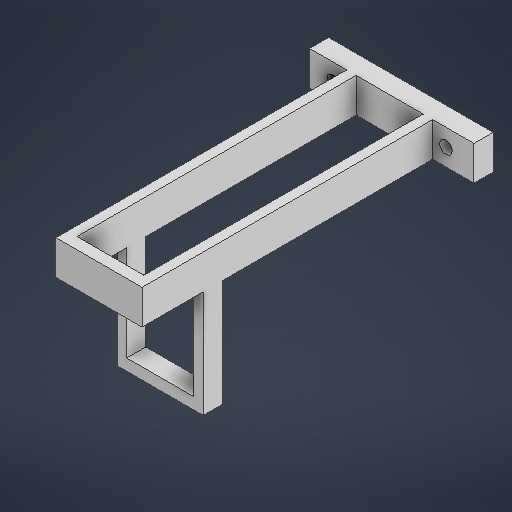
# Autodesk Inventor part: Batteryholder1
Saved by Autodesk Inventor 2026.1 (Build 301233020, 233B)
## iProperties
Created: 2025-12-01
Part Number: Batteryholder1
Material: Generic
Document SubType Name: Modeling
Designer: osama
Density: 1 g/cm^3
Appearance: Default
Author: osama
Autodesk Inventor part; units mm, degrees
ref_plane "YZ Plane" through (0, 0, 0) normal (1, 0, 0) x (0, 1, 0)
ref_plane "XZ Plane" through (0, 0, 0) normal (0, 1, 0) x (-1, 0, 0)
ref_plane "XY Plane" through (0, 0, 0) normal (0, 0, 1) x (1, 0, 0)
sketch "Sketch1" plane through (0, 0, 0) normal (0, 0, 1) x (1, 0, 0)
  line L0 (0, 0) -> (43, 0)
  line L1 (43, 0) -> (43, 9)
  line L2 (43, 9) -> (0, 9)
  line L3 (0, 9) -> (0, 0)
  dimension "d0" = 43
  dimension "d1" = 9
  constraints: 8 end point, 2 parallel, 1 horizontal, 1 perpendicular
  measures "d0" distance of L2.end L1.end
  measures "d1" distance of L1.end L0.end
extrude "Extrusion1" add sketch "Sketch1" along normal blind 5
sketch "Sketch2" plane through (0, 0, 5) normal (0, 0, 1) x (1, 0, 0)
  line L0 (43, 0) -> (43, 9) projected
  line L1 (43, 9) -> (0, 9) projected
  point P0 (0, 0)
  point P1 (35.7, 4.5)
  point P2 (6.2, 4.5)
  dimension "d11" = 7.3
  dimension "d12" = 29.5
  dimension "d13" = 4.5
  dimension "d14" = 4.5
  measures "d11" distance from line of point (35.7, 4.5) L0
  measures "d12" distance of point (35.7, 4.5) point (6.2, 4.5)
  measures "d13" distance from line of L1 point (6.2, 4.5)
  measures "d14" distance from line of L1 point (35.7, 4.5)
hole "Hole1" at (35.7, 4.5, 5) at (6.2, 4.5, 5) direction (0, 0, -1) diameter 3.3 end through all
sketch "Sketch3" plane through (0, 0, 5) normal (0, 0, 1) x (1, 0, 0)
  line L0 (0, 0) -> (43, 0) projected
  line L1 (43, 9) -> (0, 9) projected
  line L2 (9.7, 0) -> (12.2, 0)
  line L3 (12.2, 0) -> (12.2, 9)
  line L4 (12.2, 9) -> (9.7, 9)
  line L5 (9.7, 9) -> (9.7, 0)
  line L6 (29.7, 9) -> (32.2, 9)
  line L7 (32.2, 9) -> (32.2, 0)
  line L8 (32.2, 0) -> (29.7, 0)
  line L9 (29.7, 0) -> (29.7, 9)
  circle A0 centre (35.7, 4.5) radius 1.65 projected
  point P0 (29.7, 4.5)
  point P1 (12.2, 4.5)
  point P2 (32.2, 4.5)
  point P3 (29.7, 9)
  point P4 (29.7, 0)
  point P5 (32.2, 0)
  point P6 (32.2, 9)
  point P7 (12.2, 0)
  dimension "d15" = 2.5
  dimension "d16" = 2.5
  dimension "d17" = 17.5
  dimension "d18" = 3.5
  constraints: 16 end point, 4 parallel, 4 point on line, 3 midpoint, 2 horizontal, 2 perpendicular
  measures "d15" distance of L4.end L3.end
  measures "d16" distance of L7.end L8.end
  measures "d17" distance of point (29.7, 4.5) point (12.2, 4.5)
  measures "d18" distance of A0.centre point (32.2, 4.5)
extrude "Extrusion2" add sketch "Sketch3" along normal blind 76 contours L5 L1 L3 L0 | L9 L1 L7 L0
sketch "Sketch4" plane through (0, 0, 81) normal (0, 0, 1) x (1, 0, 0)
  line L0 (12.2, 9) -> (9.7, 9) projected
  line L1 (32.2, 0) -> (9.7, 0)
  line L2 (9.7, 0) -> (9.7, 9)
  line L3 (9.7, 9) -> (32.2, 9)
  line L4 (32.2, 9) -> (32.2, 0)
  point P0 (0, 0)
  constraints: 8 end point, 2 parallel, 1 horizontal, 1 perpendicular
extrude "Extrusion3" add sketch "Sketch4" against normal blind 3
sketch "Sketch7" plane through (0, 0, 0) normal (0, -1, 0) x (1, 0, 0)
  line L0 (9.7, 60) -> (9.7, 65) projected
  line L1 (9.7, 65) -> (12.2, 65)
  line L2 (12.2, 65) -> (12.2, 60)
  line L3 (12.2, 60) -> (9.7, 60)
  line L4 (9.7, 60) -> (9.7, 65)
  line L5 (32.2, 65) -> (29.7, 65) projected
  line L6 (29.7, 65) -> (32.2, 65)
  line L7 (32.2, 65) -> (32.2, 60)
  line L8 (32.2, 60) -> (29.7, 60)
  line L9 (29.7, 60) -> (29.7, 65)
  point P0 (0, 0)
  dimension "d31" = 2.5
  dimension "d32" = 5
  constraints: 16 end point, 4 parallel, 2 horizontal, 2 perpendicular, 1 point on line
  measures "d31" distance of L2.end L3.end
  measures "d32" distance of L1.end L2.end
extrude "Extrusion6" add sketch "Sketch7" along normal blind 28
sketch "Sketch8" plane through (29.7, 0, 5) normal (-1, 0, 0) x (0, 0, 1)
  line L0 (60, 0) -> (60, -28) projected
  line L1 (60, -28) -> (55, -28)
  line L2 (55, -28) -> (55, -25)
  line L3 (55, -25) -> (60, -25)
  line L4 (60, -25) -> (60, -28)
  point P0 (-5, 0)
  dimension "d35" = 5
  dimension "d36" = 3
  constraints: 8 end point, 2 parallel, 1 horizontal, 1 perpendicular
  measures "d35" distance of L2.end L3.end
  measures "d36" distance of L1.end L2.end
extrude "Extrusion7" add sketch "Sketch8" along normal blind 18
body "Solid1"
